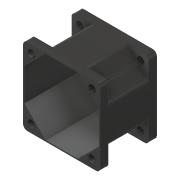
# Autodesk Inventor part: fan
Saved by Autodesk Inventor 2019 (Build 230136000, 136)
## iProperties
Created: 2020-10-21
Part Number: fan
Material: Generic
Document SubType Name: Modeling
Designer: UCLA
Density: 1 g/cm^3
Appearance: Dark Gray
Author: UCLA
Autodesk Inventor part; units mm, degrees
ref_plane "YZ Plane" through (0, 0, 0) normal (1, 0, 0) x (0, 1, 0)
ref_plane "XZ Plane" through (0, 0, 0) normal (0, 1, 0) x (-1, 0, 0)
ref_plane "XY Plane" through (0, 0, 0) normal (0, 0, 1) x (1, 0, 0)
sketch "Sketch1" plane through (0, 0, 0) normal (0, 0, 1) x (1, 0, 0)
  line L0 (19, -19) -> (-19, -19)
  line L1 (-19, -19) -> (-19, 19)
  line L2 (-19, 19) -> (19, 19)
  line L3 (19, 19) -> (19, -19)
  line L4 (19, -19) -> (-19, 19) construction
  line L5 (-19, -19) -> (19, 19) construction
  point P0 (0, 0)
  dimension "d0" = 38
  dimension "d1" = 38
  constraints: 12 end point, 2 midpoint, 2 parallel, 1 horizontal, 1 perpendicular
  measures "d0" distance of L1.end L2.end
  measures "d1" distance of L0.end L1.end
extrude "Extrusion1" add sketch "Sketch1" along normal blind 4
sketch "Sketch2" plane through (0, 0, 4) normal (0, 0, 1) x (1, 0, 0)
  line L0 (19, 19) -> (-19, 19) projected
  line L1 (-19, 19) -> (-19, -19) projected
  line L2 (8.547, -19) -> (-8.547, -19)
  line L3 (-19, -8.547) -> (-19, 8.547)
  line L4 (-8.547, 19) -> (8.547, 19)
  line L5 (19, 8.547) -> (19, -8.547)
  line L6 (19, -19) -> (-19, 19) construction
  line L7 (-19, -19) -> (19, 19) construction
  line L8 (19, 6.0309) -> (19, -12.9361)
  line L9 (-19, 8.547) -> (-8.547, 19)
  line L10 (8.547, 19) -> (19, 8.547)
  line L11 (19, -8.547) -> (8.547, -19)
  line L12 (-8.547, -19) -> (-19, -8.547)
  point P0 (0, 0)
  dimension "d16" = 38
  dimension "d17" = 38
  dimension "d18" = 10.453
  dimension "d19" = 10.453
  dimension "d20" = 10.453
  dimension "d21" = 10.453
  dimension "d22" = 10.453
  dimension "d23" = 10.453
  dimension "d24" = 10.453
  dimension "d25" = 10.453
  constraints: 22 end point, 9 point on line, 2 midpoint, 2 parallel, 1 horizontal, 1 perpendicular
  measures "d16" distance of L6.end L7.end
  measures "d17" distance of L7.start L6.end
  measures "d18" distance of L3.end L6.end
  measures "d19" distance of L4.start L6.end
  measures "d20" distance of L4.end L7.end
  measures "d21" distance of L5.start L7.end
  measures "d22" distance of L5.end L6.start
  measures "d23" distance of L2.start L6.start
  measures "d24" distance of L2.end L7.start
  measures "d25" distance of L3.start L7.start
extrude "Extrusion2" add sketch "Sketch2" along normal blind 20 contours L10 L5 L11 L2 L12 L1 L9 L0
sketch "Sketch3" plane through (0, 0, 24) normal (0, 0, 1) x (1, 0, 0)
  line L0 (19, 19) -> (-19, 19) projected
  line L1 (19, -19) -> (-19, -19)
  line L2 (-19, -19) -> (-19, 19)
  line L3 (-19, 19) -> (19, 19)
  line L4 (19, 19) -> (19, -19)
  line L5 (19, -19) -> (-19, 19) construction
  line L6 (-19, -19) -> (19, 19) construction
  point P0 (0, 0)
  constraints: 12 end point, 2 midpoint, 2 parallel, 1 horizontal, 1 perpendicular
extrude "Extrusion3" add sketch "Sketch3" along normal blind 4
sketch "Sketch5" plane through (0, 0, 28) normal (0, 0, 1) x (1, 0, 0)
  line L0 (8, -18.5) -> (-8, -18.5)
  line L1 (-18.5, -8) -> (-18.5, 8)
  line L2 (-8, 18.5) -> (8, 18.5)
  line L3 (18.5, 8) -> (18.5, -8)
  line L4 (18.5, -18.5) -> (-18.5, 18.5) construction
  line L5 (-18.5, -18.5) -> (18.5, 18.5) construction
  line L6 (-18.5, 8) -> (-8, 18.5)
  line L7 (8, 18.5) -> (18.5, 8)
  line L8 (18.5, -8) -> (8, -18.5)
  line L9 (-18.5, -8) -> (-8, -18.5)
  point P0 (0, 0)
  dimension "d27" = 37
  dimension "d28" = 37
  dimension "d29" = 10.5
  dimension "d30" = 10.5
  dimension "d31" = 10.5
  dimension "d32" = 10.5
  dimension "d33" = 10.5
  dimension "d34" = 10.5
  dimension "d35" = 10.5
  dimension "d36" = 10.5
  constraints: 20 end point, 8 point on line, 2 midpoint, 2 parallel, 1 horizontal, 1 perpendicular
  measures "d27" distance of L4.end L5.end
  measures "d28" distance of L5.start L4.end
  measures "d29" distance of L1.end L4.end
  measures "d30" distance of L2.start L4.end
  measures "d31" distance of L2.end L5.end
  measures "d32" distance of L3.start L5.end
  measures "d33" distance of L3.end L4.start
  measures "d34" distance of L0.start L4.start
  measures "d35" distance of L1.start L5.start
  measures "d36" distance of L0.end L5.start
extrude "Extrusion5" cut sketch "Sketch5" against normal blind 28
fillet "Fillet2" radius 2 16 edges at (19, 19, 26) (19, 19, 2) (-19, 19, 26) (-19, 19, 2) (-19, -19, 26) (-19, -19, 2) (19, -19, 26) (19, -19, 2) (19, -8.547, 14) (8.547, -19, 14) (-8.547, -19, 14) (-19, -8.547, 14) (-19, 8.547, 14) (-8.547, 19, 14) (8.547, 19, 14) (19, 8.547, 14)
sketch "Sketch6" plane through (0, 0, 28) normal (0, 0, 1) x (1, 0, 0)
  line L0 (-15, -15) -> (15, -15) construction
  line L1 (15, -15) -> (15, 15) construction
  line L2 (15, 15) -> (-15, 15) construction
  line L3 (-15, 15) -> (-15, -15) construction
  line L4 (-15, -15) -> (15, 15) construction
  line L5 (15, -15) -> (-15, 15) construction
  circle A0 centre (15, 15) radius 1.85
  circle A1 centre (15, -15) radius 1.85
  circle A2 centre (-15, -15) radius 1.85
  circle A3 centre (-15, 15) radius 1.85
  point P0 (0, 0)
  dimension "d40" = 30
  dimension "d41" = 30
  dimension "d42" = 3.7
  dimension "d43" = 3.7
  dimension "d44" = 3.7
  dimension "d45" = 3.7
  constraints: 12 end point, 4 centre point, 4 coincident, 2 midpoint, 2 parallel, 1 horizontal, 1 perpendicular
  measures "d40" distance of L2.end L1.end
  measures "d41" distance of L1.end L0.end
  measures "d42" diameter of A0
  measures "d43" diameter of A1
  measures "d44" diameter of A2
  measures "d45" diameter of A3
extrude "Extrusion6" cut sketch "Sketch6" against normal blind 28
equation "\"d19\" = d18"
equation "\"d20\" = d18"
equation "\"d21\" = d20"
equation "\"d22\" = d18"
equation "\"d23\" = d22"
equation "\"d24\" = d18"
equation "\"d25\" = d24"
equation "\"d30\" = d29"
equation "\"d31\" = d29"
equation "\"d32\" = d31"
equation "\"d33\" = d29"
equation "\"d34\" = d33"
equation "\"d35\" = d29"
equation "\"d36\" = d35"
body "Solid1"
